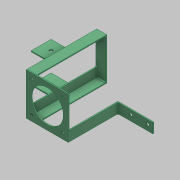
# Autodesk Inventor part: MotorSupport
Saved by Autodesk Inventor 2018 (Build 220112000, 112)
## iProperties
Created: 2019-07-12
Part Number: MotorSupport
Material: Generic
Document SubType Name: Modeling
Designer: mkivekas
Density: 1 g/cm^3
Appearance: Smooth - Dark Sea Green
Author: mkivekas
Autodesk Inventor part; units mm, degrees
ref_plane "YZ Plane" through (0, 0, 0) normal (1, 0, 0) x (0, 1, 0)
ref_plane "XZ Plane" through (0, 0, 0) normal (0, 1, 0) x (-1, 0, 0)
ref_plane "XY Plane" through (0, 0, 0) normal (0, 0, 1) x (1, 0, 0)
sketch "Sketch1" plane through (0, 0, 0) normal (0, 1, 0) x (-1, 0, 0)
  line L0 (-21.15, -21.15) -> (21.15, -21.15)
  line L1 (21.15, -21.15) -> (21.15, 21.15)
  line L2 (21.15, 21.15) -> (-21.15, 21.15)
  line L3 (-21.15, 21.15) -> (-21.15, -21.15)
  line L4 (-21.15, -21.15) -> (21.15, 21.15) construction
  line L5 (21.15, -21.15) -> (-21.15, 21.15) construction
  circle A0 centre (0, 0) radius 16.15
  point P0 (15.59, 15.59)
  point P1 (-15.59, 15.59)
  point P2 (-15.59, -15.59)
  point P3 (15.59, -15.59)
  dimension "d0" = 42.3
  dimension "d1" = 42.3
  dimension "d2" = 5
  dimension "d3" = 5.56
  dimension "d6" = 360
  dimension "d121" = 5.56
  constraints: 12 end point, 2 midpoint, 2 parallel, 1 centre point, 1 coincident, 1 horizontal, 1 perpendicular, 1 point on line, 5 other
  measures "d0" distance of L1.end L2.end
  measures "d1" distance of L0.end L1.end
  measures "d2" distance edge to line of A0 L2
  measures "d3" distance from line of L1 point (15.59, 15.59)
  measures "d121" distance from line of L2 point (15.59, 15.59)
extrude "Extrusion1" add sketch "Sketch1" along normal blind 1
hole "Hole1" at (-15.59, 0, 15.59) at (15.59, 0, 15.59) at (15.59, 0, -15.59) at (-15.59, 0, -15.59) direction (0, 1, 0) diameter 2.459 depth 8.8 tip angle 118 thread size "M3x0.5" class "6H" standard "ISO Metric profile"
sketch "Sketch3" plane through (0, 1, 0) normal (0, 1, 0) x (1, 0, 0)
  line L0 (21.15, -21.15) -> (21.15, 21.15) projected
  line L1 (21.15, 15.8) -> (20.15, 15.8)
  line L2 (20.15, 15.8) -> (20.15, 21.15)
  line L3 (20.15, 21.15) -> (21.15, 21.15)
  line L4 (21.15, 21.15) -> (21.15, 15.8)
  line L5 (21.15, 15.8) -> (20.15, 15.8)
  line L6 (20.15, 15.8) -> (20.15, 11.15)
  line L7 (20.15, 11.15) -> (21.15, 11.15)
  line L8 (21.15, 11.15) -> (21.15, 15.8)
  line L9 (21.15, 21.15) -> (-21.15, 21.15) projected
  point P0 (0, 0)
  dimension "d27" = 15.8
  dimension "d28" = 1
  dimension "d29" = 0
  dimension "d30" = 10
  dimension "d36" = 5.35
  constraints: 16 end point, 4 parallel, 2 horizontal, 2 perpendicular, 1 point on line
  measures "d27" vertical distance of L1.end point (0, 0)
  measures "d28" distance between parallel lines of L0 L2
  measures "d29" distance from line of L3.end L9
  measures "d30" vertical distance of L7.end L2.end
  measures "d36" distance of L1.end L2.end
extrude "Extrusion3" add sketch "Sketch3" along normal blind 50
sketch "Sketch4" plane through (21.15, 0, 21.15) normal (1, 0, 0) x (0, 0, -1)
  line L0 (32.3, 1) -> (32.3, 51) projected
  line L1 (42.3, 1) -> (42.3, 51) projected
  line L2 (32.3, 51) -> (42.3, 51)
  line L3 (42.3, 51) -> (42.3, 50)
  line L4 (42.3, 50) -> (32.3, 50)
  line L5 (32.3, 50) -> (32.3, 51)
  point P0 (21.15, 0)
  dimension "d33" = 1
  constraints: 8 end point, 2 parallel, 1 horizontal, 1 perpendicular, 1 point on line
  measures "d33" distance between parallel lines of L2 L4
extrude "Extrusion4" add sketch "Sketch4" along normal blind 35
sketch "Sketch5" plane through (21.15, 50, -21.15) normal (0, -1, 0) x (1, 0, 0)
  line L0 (0, 0) -> (35, 0) projected
  line L1 (0, 0) -> (0, 10) projected
  point P0 (-21.15, 21.15)
  point P1 (12.85, 5.45)
  point P2 (29.85, 5.45)
  dimension "d37" = 5.45
  dimension "d39" = 17
  dimension "d120" = 34
  constraints: 1 horizontal alignment
  measures "d37" distance from line of L0 point (12.85, 5.45)
  measures "d39" distance of point (29.85, 5.45) point (12.85, 5.45)
  measures "d120" horizontal distance of point (12.85, 5.45) point (-21.15, 21.15)
hole "Hole2" at (34, 50, -15.7) at (51, 50, -15.7) direction (0, 1, 0) diameter 3.242 depth 11.8 tip angle 118 thread size "M4x0.7" class "6H" standard "ISO Metric profile"
sketch "Sketch7" plane through (0, 1, 0) normal (0, 1, 0) x (1, 0, 0)
  line L0 (21.15, 21.15) -> (-21.15, 21.15) projected
  line L1 (-21.15, 21.15) -> (-11.15, 21.15)
  line L2 (-11.15, 21.15) -> (-11.15, 20.15)
  line L3 (-11.15, 20.15) -> (-21.15, 20.15)
  line L4 (-21.15, 20.15) -> (-21.15, 21.15)
  point P0 (0, 0)
  dimension "d47" = 10
  dimension "d48" = 1
  constraints: 8 end point, 2 parallel, 1 horizontal, 1 perpendicular
  measures "d47" distance of L2.end L3.end
  measures "d48" distance of L3.end L0.end
extrude "Extrusion5" add sketch "Sketch7" along normal blind 70
sketch "Sketch8" plane through (-21.15, 0, -21.15) normal (-1, 0, 0) x (0, 0, 1)
  line L0 (0, 1) -> (0, 71) projected
  line L1 (0, 71) -> (42.3, 71)
  line L2 (42.3, 71) -> (42.3, 70)
  line L3 (42.3, 70) -> (0, 70)
  line L4 (0, 70) -> (0, 71)
  point P0 (21.15, 0)
  dimension "d51" = 1
  dimension "d52" = 42.3
  constraints: 8 end point, 2 parallel, 1 horizontal, 1 perpendicular
  measures "d51" distance of L1.end L2.end
  measures "d52" distance of L0.end L1.end
extrude "Extrusion6" add sketch "Sketch8" against normal blind 10
sketch "Sketch10" plane through (0, 71, 0) normal (0, 1, 0) x (1, 0, 0)
  line L0 (-11.15, 21.15) -> (-21.15, 21.15) projected
  line L1 (-21.15, 21.15) -> (-21.15, -21.15) projected
  point P0 (0, 0)
  point P1 (-18.9, 6.7)
  point P2 (-18.9, -11.3)
  dimension "d57" = 14.45
  dimension "d58" = 2.25
  dimension "d74" = 18
  measures "d57" distance from line of point (-18.9, 6.7) L0
  measures "d58" distance from line of L1 point (-18.9, 6.7)
  measures "d74" distance of point (-18.9, 6.7) point (-18.9, -11.3)
hole "Hole3" at (-18.9, 71, -6.7) at (-18.9, 71, 11.3) direction (0, -1, 0) diameter 2.013 depth 7.6 tip angle 118 thread size "M2.5x0.45" class "6H" standard "ISO Metric profile"
sketch "Sketch11" plane through (0, 1, 0) normal (0, 1, 0) x (1, 0, 0)
  line L0 (-11.15, 20.15) -> (-21.15, 20.15) projected
  line L1 (-21.15, 20.15) -> (-20.15, 20.15)
  line L2 (-20.15, 20.15) -> (-20.15, 11.15)
  line L3 (-20.15, 11.15) -> (-21.15, 11.15)
  line L4 (-21.15, 11.15) -> (-21.15, 20.15)
  line L5 (-11.15, -21.1519) -> (-21.15, -21.1519)
  line L6 (-21.15, -21.1519) -> (-21.15, -13.1519)
  line L7 (-21.15, 20.15) -> (-21.15, -21.15) projected
  line L8 (-21.15, -13.1519) -> (-20.15, -13.1519)
  line L9 (-20.15, -13.1519) -> (-20.15, -20.1519)
  line L10 (-20.15, -20.1519) -> (-11.15, -20.1519)
  line L11 (-11.15, -20.1519) -> (-11.15, -21.1519)
  line L12 (-21.15, -21.15) -> (21.15, -21.15) projected
  point P0 (0, 0)
  dimension "d66" = 1
  dimension "d67" = 9
  dimension "d68" = 1
  dimension "d69" = 1
  dimension "d70" = 10
  dimension "d71" = 8
  constraints: 20 end point, 4 perpendicular, 3 parallel, 2 horizontal, 1 point on line
  measures "d66" distance of L2.end L3.end
  measures "d67" distance of L1.end L2.end
  measures "d68" distance between parallel lines of L6 L9
  measures "d69" distance between parallel lines of L5 L10
  measures "d70" distance of L7.end L5.start
  measures "d71" distance of L5.end L6.end
extrude "Extrusion7" add sketch "Sketch11" along normal blind 70
sketch "Sketch12" plane through (-21.15, 0, -21.15) normal (-1, 0, 0) x (0, 0, 1)
  line L0 (34.3019, 1) -> (34.3019, 70) projected
  line L1 (10, 1) -> (10, 50) projected
  line L2 (0, 0) -> (42.3, 0) projected
  line L3 (7, 45) -> (6, 45)
  line L4 (6, 45) -> (6, 25)
  line L5 (6, 25) -> (7, 25)
  line L6 (7, 25) -> (7, 45)
  line L7 (35.3019, 45) -> (36.3019, 45)
  line L8 (36.3019, 45) -> (36.3019, 25)
  line L9 (36.3019, 25) -> (35.3019, 25)
  line L10 (35.3019, 25) -> (35.3019, 45)
  point P0 (21.15, 0)
  point P1 (34.3019, 25)
  point P2 (10, 25)
  point P3 (32.4996, 66.5)
  dimension "d78" = 25
  dimension "d90" = 1
  dimension "d91" = 1
  dimension "d92" = 20
  dimension "d93" = 20
  dimension "d94" = 25
  dimension "d95" = 25
  dimension "d96" = 3
  dimension "d97" = 1
  constraints: 16 end point, 4 parallel, 2 horizontal, 2 perpendicular, 1 point on line, 2 other
  measures "d78" distance from line of L2 point (10, 25)
  measures "d90" distance of L3.start L3.end
  measures "d91" distance of L7.start L7.end
  measures "d92" distance of L3.end L4.end
  measures "d93" distance of L7.end L8.end
  measures "d94" distance from line of L2 L4.end
  measures "d95" distance from line of L2 L9.end
  measures "d96" distance between parallel lines of L1 L6
extrude "Extrusion8" add sketch "Sketch12" along normal blind 20
sketch "Sketch14" plane through (-21.15, 25, -15.15) normal (0, 0, -1) x (-1, 0, 0)
  line L0 (0, 0) -> (0, 20) projected
  line L1 (20, 20) -> (20, 0) projected
  line L2 (0, 20) -> (20, 0)
  line L3 (20, 0) -> (20, 20)
  line L4 (20, 20) -> (0, 0)
  point P0 (-21.15, -25)
  point P1 (10, 10)
  constraints: 6 end point, 1 collinear, 1 midpoint, 1 perpendicular
hole "Hole5" at (-31.15, 35, -15.15) direction (0, 0, 1) diameter 3.242 depth 50 tip angle 118 thread size "M4x0.7" class "6H" standard "ISO Metric profile"
chamfer "Chamfer1" distance 1 angle 45 4 edges at (-21.15, 35, 14.1519) (-21.15, 45, 14.6519) (-21.15, 25, 14.6519) (-21.15, 35, 15.1519)
chamfer "Chamfer2" distance 1 angle 45 4 edges at (-21.15, 35, -14.15) (-21.15, 25, -14.65) (-21.15, 35, -15.15) (-21.15, 45, -14.65)
chamfer "Chamfer3" distance 1 angle 45 1 edges at (21.15, 50, -16.15)
chamfer "Chamfer4" distance 1 angle 45 6 edges at (-15.65, 70, -20.15) (-20.15, 70, -15.65) (-20.65, 70, -11.15) (-20.65, 70, 13.1519) (-20.15, 70, 16.6519) (-15.65, 70, 20.1519)
chamfer "Chamfer5" distance 1 angle 45 8 edges at (-11.15, 1, 20.6509) (-11.15, 1, -20.65) (-15.65, 1, 20.1519) (-20.15, 1, 16.6519) (-20.65, 1, 13.1519) (-20.15, 1, -15.65) (-15.65, 1, -20.15) (-20.65, 1, -11.15)
sketch "Sketch2" plane through (0, 1, 0) normal (0, 1, 0) x (1, 0, 0)
  line L0 (-21.15, -21.15) -> (21.15, -21.15) projected
  line L1 (-11.15, -21.15) -> (-11.15, -20.15)
  line L2 (-11.15, -20.15) -> (-20.15, -20.15)
  line L3 (-20.15, -20.15) -> (-20.15, -11.15)
  line L4 (-20.15, -11.15) -> (-20.5996, -11.15)
  line L5 (-20.5996, -11.15) -> (-21.15, -11.15)
  line L6 (-21.15, 21.15) -> (-21.15, -21.15) projected
  line L7 (-21.15, -11.15) -> (-21.15, -21.15)
  line L8 (-21.15, -21.15) -> (-11.15, -21.15)
  line L9 (21.15, -11.15) -> (20.15, -11.15)
  line L10 (20.15, -11.15) -> (20.15, -20.15)
  line L11 (20.15, -20.15) -> (11.15, -20.15)
  line L12 (11.15, -20.15) -> (11.15, -20.5996)
  line L13 (11.15, -20.5996) -> (11.15, -21.15)
  line L14 (11.15, -21.15) -> (21.15, -21.15)
  line L15 (21.15, -21.15) -> (21.15, -11.15)
  line L16 (11.15, 21.15) -> (11.15, 20.15)
  line L17 (11.15, 20.15) -> (20.15, 20.15)
  line L18 (20.15, 20.15) -> (20.15, 11.15)
  line L19 (20.15, 11.15) -> (20.5996, 11.15)
  line L20 (20.5996, 11.15) -> (21.15, 11.15)
  line L21 (21.15, 11.15) -> (21.15, 21.15)
  line L22 (21.15, 21.15) -> (11.15, 21.15)
  line L23 (-21.15, 11.15) -> (-20.15, 11.15)
  line L24 (-20.15, 11.15) -> (-20.15, 20.15)
  line L25 (-20.15, 20.15) -> (-11.15, 20.15)
  line L26 (-11.15, 20.15) -> (-11.15, 20.5996)
  line L27 (-11.15, 20.5996) -> (-11.15, 21.15)
  line L28 (-11.15, 21.15) -> (-21.15, 21.15)
  line L29 (-21.15, 21.15) -> (-21.15, 11.15)
  point P0 (0, 0)
  dimension "d17" = 10
  dimension "d18" = 10
  dimension "d19" = 1
  dimension "d20" = 1
  dimension "d23" = 360
  constraints: 56 end point, 4 perpendicular, 2 collinear, 1 horizontal, 1 point on line, 57 other
  measures "d17" distance from line of L1 L0.start
  measures "d18" distance from line of L4 L0.start
  measures "d19" distance between parallel lines of L0 L2
  measures "d20" distance between parallel lines of L6 L3
body "Solid1"
